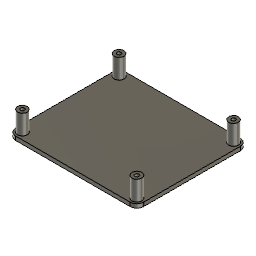
PiHalterung (Autodesk Fusion 360 design; units mm, degrees)
part number: 2025-12-13-20-25-32-821
Autodesk Fusion 360 part; units mm, degrees
note: some values were not read from the file. Set by a fixed rule: which sketch regions a step uses.
sketch "Skizze1" plane through (0, 0, 0) normal (0, 0, 1) x (1, 0, 0)
  line L0 (0, 0) -> (95, 0)
  line L1 (95, 0) -> (95, 66)
  line L2 (95, 66) -> (0, 66)
  line L3 (0, 66) -> (0, 0)
  line L4 (47.5, 0) -> (47.5, 66) construction
  line L5 (0, 33) -> (95, 33) construction
  line L6 (90, 61) -> (5, 61)
  line L7 (5, 61) -> (5, 5)
  line L8 (5, 5) -> (90, 5)
  line L9 (90, 5) -> (90, 61)
  line L10 (90, 61) -> (5, 5) construction
  line L11 (5, 61) -> (90, 5) construction
  line L12 (5, 61) -> (8.5, 61)
  line L13 (8.5, 61) -> (8.5, 57.5)
  line L14 (8.5, 57.5) -> (5, 57.5)
  line L15 (5, 57.5) -> (5, 61)
  circle A0 centre (8.5, 57.5) radius 2.5
  line L16 (5, 5) -> (8.5, 5)
  line L17 (8.5, 5) -> (8.5, 8.5)
  line L18 (8.5, 8.5) -> (5, 8.5)
  line L19 (5, 8.5) -> (5, 5)
  circle A1 centre (8.5, 8.5) radius 2.5
  line L20 (8.5, 8.5) -> (66.5, 8.5)
  circle A2 centre (66.5, 8.5) radius 2.5
  line L21 (8.5, 57.5) -> (66.5, 57.5)
  circle A3 centre (66.5, 57.5) radius 2.5
  point P0 (47.5, 33)
  dimension "d1" = 95
  dimension "d2" = 66
  dimension "d3" = 85
  dimension "d4" = 56
  dimension "d5" = 3.5
  dimension "d6" = 3.5
  dimension "d7" = 5
  dimension "d8" = 3.5
  dimension "d9" = 3.5
  dimension "d10" = 5
  dimension "d11" = 58
  dimension "d12" = 5
  dimension "d13" = 58
  dimension "d14" = 5
  constraint horizontal L0
  constraint vertical L1
  constraint horizontal L2
  constraint vertical L3
  constraint coincident L0.start L3.end
  constraint midpoint L0 L4.start
  constraint midpoint L2 L4.end
  constraint midpoint L3 L5.start
  constraint midpoint L1 L5.end
  constraint horizontal L6
  constraint perpendicular L6 L7
  constraint parallel L6 L8
  constraint parallel L7 L9
  constraint coincident L10 P0
  constraint coincident L11 P0
  constraint midpoint L4 P0
  constraint horizontal L12
  constraint vertical L13
  constraint horizontal L14
  constraint vertical L15
  constraint coincident L13.end L14.start
  constraint horizontal L16
  constraint vertical L17
  constraint horizontal L18
  constraint vertical L19
  constraint coincident L17.end L18.start
  constraint horizontal L20
  constraint coincident L20.end A2.centre
  constraint perpendicular L13 L21
  constraint coincident L21.end A3.centre
  measures "d1" distance of L0.start L0.end
  measures "d2" distance of L0.start L2.end
  measures "d3" distance of L7.end L8.end
  measures "d4" distance of L6.end L7.end
  measures "d5" distance of L6.end L12.end
  measures "d6" distance of L6.end L14.end
  measures "d7" diameter of A0
  measures "d8" distance of L7.end L16.end
  measures "d9" distance of L7.end L18.end
  measures "d10" diameter of A1
  measures "d11" distance of L17.end L20.end
  measures "d12" diameter of A2
  measures "d13" distance of L13.end L21.end
  measures "d14" diameter of A3
extrude "Extrusion1" add sketch "Skizze1" along normal blind 2 contours L0 L1 L2 L3 | L6 L7 L8 L9 L13 L14 A0 L17 L18 A1 | L6 L7 L12 L13 L14 L15 A0 | L7 L8 L16 L17 L18 L19 A1
extrude "Extrusion2" add sketch "Skizze1" along normal blind 12 contours L13 A0 L21 | L13 L14 A0 | L14 A0 L21 | L17 L18 A1 | L17 A1 L20 | L18 A1 L20 | A2 | A3
sketch "Skizze2" plane through (0, 0, 12) normal (0, 0, 1) x (-1, 0, 0)
  circle A0 centre (-8.5, -57.5) radius 2.5
  circle A1 centre (-8.5, -57.5) radius 1
  dimension "d19" = 2
  constraint concentric A0 A1
  measures "d19" diameter of A1
extrude "Extrusion3" cut sketch "Skizze2" against normal blind 10 contours A1
sketch "Skizze3" plane through (0, 0, 12) normal (0, 0, 1) x (-1, 0, 0)
  circle A0 centre (-8.5, -8.5) radius 2.5
  circle A1 centre (-8.5, -8.5) radius 1
  dimension "d22" = 2
  constraint concentric A0 A1
  measures "d22" diameter of A1
extrude "Extrusion4" cut sketch "Skizze3" against normal blind 10 contours A1
sketch "Skizze4" plane through (0, 0, 12) normal (0, 0, 1) x (-1, 0, 0)
  circle A0 centre (-66.5, -8.5) radius 2.5
  circle A1 centre (-66.5, -8.5) radius 1
  dimension "d25" = 2
  constraint concentric A0 A1
  measures "d25" diameter of A1
extrude "Extrusion5" cut sketch "Skizze4" against normal blind 10 contours A1
sketch "Skizze5" plane through (0, 0, 12) normal (0, 0, 1) x (-1, 0, 0)
  circle A0 centre (-66.5, -57.5) radius 2.5
  circle A1 centre (-66.5, -57.5) radius 1
  dimension "d28" = 2
  constraint concentric A0 A1
  measures "d28" diameter of A1
extrude "Extrusion6" cut sketch "Skizze5" against normal blind 10 contours A1
extrude "Extrusion7" cut 4 faces at (8.8074, 8.4503, 2) (8.2374, 57.0304, 2) (66.1815, 58.0517, 2) (66.5787, 9.0963, 2) along direction (0, 0, -1) blind 1
sketch "Skizze6" plane through (0, 0, 2) normal (0, 0, 1) x (-1, 0, 0)
  circle A0 centre (-66.5, -57.5) radius 2.5
  circle A1 centre (-8.5, -8.5) radius 2.5
  circle A2 centre (-8.5, -57.5) radius 2.5
  circle A3 centre (-66.5, -8.5) radius 2.5
  line L0 (0, -66) -> (0, 0)
  line L1 (0, 0) -> (-95, 0)
  line L2 (-95, 0) -> (-95, -66)
  line L3 (-95, -66) -> (0, -66)
  circle A4 centre (-8.5, -57.5) radius 3.5
  circle A5 centre (-66.5, -57.5) radius 3.5
  circle A6 centre (-8.5, -8.5) radius 3.5
  dimension "d33" = 7
  dimension "d34" = 7
  dimension "d35" = 7
  constraint concentric A2 A4
  constraint concentric A0 A5
  constraint concentric A1 A6
  measures "d33" diameter of A4
  measures "d34" diameter of A5
  measures "d35" diameter of A6
extrude "Extrusion8" cut sketch "Skizze1" along normal blind 2 contours L0 L1 L2 L3
extrude "Extrusion9" cut 1 faces at (90, 23.6667, 0.6667) along direction (-1, 0, 0) blind 20
fillet "Abrundung1" radius 3.5 4 edges at (5, 5, 1) (70, 5, 1) (70, 61, 1) (5, 61, 1)
